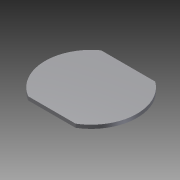
# Autodesk Inventor part: superior
Saved by Autodesk Inventor 2012 (Build 160160000, 160)
## iProperties
Created: 2013-01-02
Part Number: superior
Material: Default
Document SubType Name: Modeling
Designer: asimov
Density: 1 g/cm^3
Author: asimov
Autodesk Inventor part; units mm, degrees
ref_plane "YZ Plane" through (0, 0, 0) normal (1, 0, 0) x (0, 1, 0)
ref_plane "XZ Plane" through (0, 0, 0) normal (0, 1, 0) x (-1, 0, 0)
ref_plane "XY Plane" through (0, 0, 0) normal (0, 0, 1) x (1, 0, 0)
sketch "Sketch1" plane through (0, 0, 0) normal (0, 0, 1) x (1, 0, 0)
  line L0 (0, 31.071) -> (22.7086, 31.071)
  line L1 (0, 31.071) -> (-22.7086, 31.071)
  line L2 (0, -32.929) -> (19.9189, -32.929)
  line L3 (0, -32.929) -> (-19.9189, -32.929)
  arc A0 (-22.7086, 31.071) -> (-19.9189, -32.929) centre (0, 0) ccw
  arc A1 (19.9189, -32.929) -> (22.7086, 31.071) centre (0, 0) ccw
  dimension "d2" = 64
  constraints: 8 end point, 4 point on circle, 2 centre point, 1 coincident
  measures "d2" distance between parallel lines of L2 L0
extrude "Extrusion1" add sketch "Sketch1" along normal blind 3
body "Solid1"
